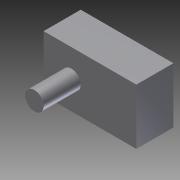
# Autodesk Inventor part: proxycimulator775
Saved by Autodesk Inventor 2011 SP1 (Build 150282100, 282)
## iProperties
Created: 2012-01-20
Part Number: proxycimulator775
Document SubType Name: Modeling
Designer: Christopher
Density: 1 g/cm^3
Author: Christopher
Autodesk Inventor part; units mm, degrees
ref_plane "YZ Plane" through (0, 0, 0) normal (1, 0, 0) x (0, 1, 0)
ref_plane "XZ Plane" through (0, 0, 0) normal (0, 1, 0) x (-1, 0, 0)
ref_plane "XY Plane" through (0, 0, 0) normal (0, 0, 1) x (1, 0, 0)
sketch "Sketch1" plane through (0, 0, 0) normal (0, 0, 1) x (1, 0, 0)
  line L0 (0, 0) -> (63.5, 0)
  line L1 (63.5, 0) -> (63.5, 38.1)
  line L2 (63.5, 38.1) -> (0, 38.1)
  line L3 (0, 38.1) -> (0, 0)
  circle A0 centre (19.05, 19.05) radius 6.35
  dimension "d0" = 63.5
  dimension "d1" = 38.1
  dimension "d4" = 19.05
  dimension "d5" = 12.7
  constraints: 8 end point, 2 parallel, 1 centre point, 1 coincident, 1 horizontal, 1 perpendicular
  measures "d0" distance of L1.end L2.end
  measures "d1" distance of L2.end L0.start
  measures "d4" distance from line of L3 point (19.05, 19.05)
  measures "d5" diameter of A0
extrude "Extrusion1" add sketch "Sketch1" against normal blind 25.4 contours L3 L2 L1 L0 | A0
extrude "Extrusion2" add sketch "Sketch1" along normal blind 25.4 contours A0
sketch "Sketch2" plane through (0, 0, -25.4) normal (0, 0, -1) x (-1, 0, 0)
  line L0 (-63.5, 0) -> (-63.5, 38.1) projected
  circle A0 centre (-44.45, 19.05) radius 8.4036
  dimension "d8" = 19.05
  constraints: 1 centre point, 1 coincident
  measures "d8" distance from line of L0 point (-44.45, 19.05)
hole "Hole1" at (44.45, 19.05, -25.4) direction (0, 0, 1) diameter 5.08 depth 7.62 tip angle 118
body "Solid1"
